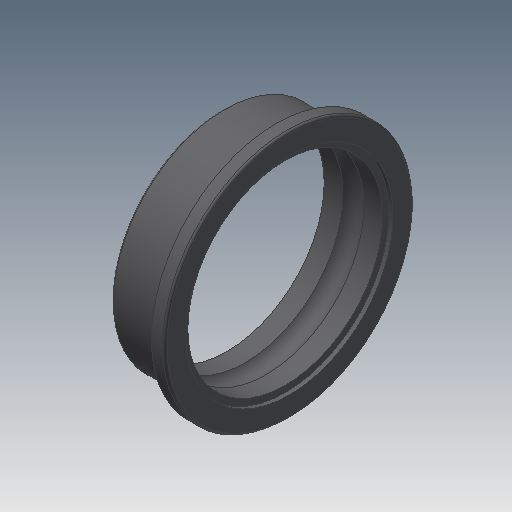
# Autodesk Inventor part: MF106ZZ1 Outer Ring
Saved by Autodesk Inventor 2019.4 (Build 234330000, 330)
## iProperties
Category: PARTsolutions
Company: NSK_RB
Created: 2019-11-13
Part Number: MF106ZZ1 Outer Ring
Material: 一般
Catalog Web Link: www.cadenas.de
Description: shielded_type_zz_zzs_OR-
Vendor: NSK_RB
Document SubType Name: Modeling
Designer: psadmin
Manufacturer: NSK_RB
Mass: 0.0599707 g
Surface Area: 2.58339 cm^2
Volume: 0.0599707 cm^3
Density: 1 g/cm^3
Appearance: PSOLRGB-128-128-128
PSOL_IDENT_0: {$CADENAS_DATA\23d-libs\nsk_rb\roller_bearings\deep_groove_bb\exstra_small_miniatur_bb\metric_design
PSOL_IDENT_1: _with_flange\shielded_type_zz_zzs_or1.prj},196 {VTYP=3D},{NB=MF106ZZ1 Outer Ring},{LINA=MF106ZZ1 Out
PSOL_IDENT_2: er Ring},{NN=shielded_type_zz_zzs_OR},{DATE=16.01.2019 01:41:14},{GEOMDATE=04.01.2008 00:00:00},{VER
PSOL_IDENT_3: SION=},{LINEID=580},{WBVAR=},{WBNUMERIC=}  {NB=MF106ZZ1 Outer Ring},{LINA=MF106ZZ1 Outer Ring},{KT=D
PSOL_IDENT_4: UMMY},{IDNR=},{STAN=},{ORDER=MF106ZZ1},{SD=6.0},{X=6.0},{D=10},{DD=10},{DD1=0.0},{D2=11.2},{DD2=11.2
PSOL_IDENT_5: },{B=0.0},{B1=3.0},{CC1=0.0},{C2=0.6},{CC2=0.6},{R=0.00},{R1=0.10},{DI1=7.00},{DI2=7.00},{SDE1=8.75}
PSOL_IDENT_6: ,{SDE2=9.31},{CR1=495},{COR1=218},{CR2=51},{COR2=22.0},{LG=45000},{LO=53000},{DA=0.0},{DB=7.0},{RA=0
PSOL_IDENT_7: .00},{RB=0.10},{MASS=0.77},{SC=1}
NN: shielded_type_zz_zzs_OR
NB: MF106ZZ1 Outer Ring
NBSYN: $ORDER. Outer Ring
LINA: MF106ZZ1 Outer Ring
ORDER: MF106ZZ1
SD: 6
X: 6
D: 10
DD: 10
DD1: 0
D2: 11.2
DD2: 11.2
B: 0
B1: 3
CC1: 0
C2: 0.6
CC2: 0.6
R: 0
R1: 0.1
DI1: 7
DI2: 7
SDE1: 8.75
SDE2: 9.31
CR1: 495
COR1: 218
CR2: 51
COR2: 22
LG: 45000
LO: 53000
DA: 0
DB: 7
RA: 0
RB: 0.1
MASS: 0.77
SC: 1
SUPPLIER: NSK_RB
ARTICLENO: MF106ZZ1 Outer Ring
BOMINFO: MF106ZZ1 Outer Ring
CREATOR: CADENAS GmbH
Title: MF106ZZ1 Outer Ring
Author: Cadenas PARTsolutions
Autodesk Inventor part; units mm, degrees
sketch "Sketch_1" plane through (0, 0, 0) normal (0, 0, 1) x (1, 0, 0)
  line L0 (3, 0) -> (0, 0)
  line L1 (0, 4.655) -> (0.1875, 4.655)
  line L2 (0.1875, 4.655) -> (0.1875, 4.375)
  line L3 (0.1875, 4.375) -> (1.0316, 4.375)
  arc A0 (1.9684, 4.375) -> (1.0316, 4.375) centre (1.5, 4) ccw
  line L4 (1.9684, 4.375) -> (2.8125, 4.375)
  line L5 (2.8125, 4.375) -> (2.8125, 4.655)
  line L6 (2.8125, 4.655) -> (3, 4.655)
  line L7 (3, 4.655) -> (3, 5.5)
  arc A1 (3, 5.5) -> (2.9, 5.6) centre (2.9, 5.5) ccw
  line L8 (2.9, 5.6) -> (2.4, 5.6)
  line L9 (2.4, 5.6) -> (2.4, 5)
  line L10 (2.4, 5) -> (0.1, 5)
  arc A2 (0.1, 5) -> (0, 4.9) centre (0.1, 4.9) ccw
  line L11 (0, 4.9) -> (0, 4.655)
  constraints: 24 end point, 6 point on circle, 3 centre point
revolve "Revolution1" add sketch "Sketch_1" angle 360 about axis through (3, 0, 0) along (1, 0, 0)
ref_plane "ip_st_1_XY" through (0, 0, 0) normal (1, 0, 0) x (0, 0, -1)
ref_plane "ip_st_1_YZ" through (0, 0, 0) normal (0, 0, -1) x (0, 1, 0)
ref_plane "ip_st_1_ZX" through (0, 0, 0) normal (0, 1, 0) x (1, 0, 0)
ref_plane "ip_st_2_XY" through (2.8125, 0, 0) normal (-1, 0, 0) x (0, 0, -1)
ref_plane "ip_st_2_YZ" through (2.8125, 0, 0) normal (0, 0, -1) x (0, -1, 0)
ref_plane "ip_st_2_ZX" through (2.8125, 0, 0) normal (0, -1, 0) x (-1, 0, 0)
body "Solid1"
